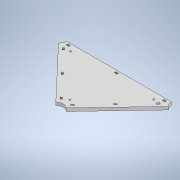
# Autodesk Inventor part: aab_face
Saved by Autodesk Inventor 2020 (Build 240168000, 168)
## iProperties
Created: 2019-09-26
Part Number: aab_face
Material: Generic
Document SubType Name: Modeling
Designer: fabrizio
Density: 1 g/cm^3
Appearance: Default
Author: fabrizio
Autodesk Inventor part; units mm, degrees
ref_plane "YZ Plane" through (0, 0, 0) normal (1, 0, 0) x (0, 1, 0)
ref_plane "XZ Plane" through (0, 0, 0) normal (0, 1, 0) x (-1, 0, 0)
ref_plane "XY Plane" through (0, 0, 0) normal (0, 0, 1) x (1, 0, 0)
sketch "Sketch1" plane through (0, 0, 0) normal (0, 1, 0) x (-1, 0, 0)
  arc A0 (10, 0) -> (6.8806, 7.2566) centre (0, 0) ccw
  arc A1 (151.2194, 7.2566) -> (148.1, 0.0154) centre (158.1, 0) ccw
  circle A2 centre (79.05, 64.475) radius 1
  circle A3 centre (133.744, 8.9222) radius 1
  circle A4 centre (24.356, 8.9222) radius 1
  line L0 (6.8806, 7.2566) -> (72.1694, 76.1134)
  line L1 (85.9306, 76.1134) -> (151.2194, 7.2566)
  line L2 (148.1, 0.0154) -> (10, 0)
  arc A5 (72.1694, 76.1134) -> (85.9306, 76.1134) centre (79.05, 83.37) ccw
  line L3 (14.0684, 2.4018) -> (17.5684, 2.4018)
  line L4 (17.5684, 2.4018) -> (17.5684, 4.4018)
  line L5 (17.5684, 4.4018) -> (14.0684, 4.4018)
  line L6 (14.0684, 4.4018) -> (14.0684, 2.4018)
  line L7 (77.3084, 2.4018) -> (80.8084, 2.4018)
  line L8 (80.8084, 2.4018) -> (80.8084, 4.4018)
  line L9 (80.8084, 4.4018) -> (77.3084, 4.4018)
  line L10 (77.3084, 4.4018) -> (77.3084, 2.4018)
  line L11 (140.5484, 2.4018) -> (144.0484, 2.4018)
  line L12 (144.0484, 2.4018) -> (144.0484, 4.4018)
  line L13 (144.0484, 4.4018) -> (140.5484, 4.4018)
  line L14 (140.5484, 4.4018) -> (140.5484, 2.4018)
  line L15 (16.2824, 8.7713) -> (18.6906, 11.3111)
  line L16 (18.6906, 11.3111) -> (17.2392, 12.6872)
  line L17 (17.2392, 12.6872) -> (14.831, 10.1474)
  line L18 (14.831, 10.1474) -> (16.2824, 8.7713)
  line L19 (43.688, 37.6746) -> (46.0962, 40.2145)
  line L20 (46.0962, 40.2145) -> (44.6449, 41.5906)
  line L21 (44.6449, 41.5906) -> (42.2367, 39.0508)
  line L22 (42.2367, 39.0508) -> (43.688, 37.6746)
  line L23 (71.0937, 66.578) -> (73.5019, 69.1178)
  line L24 (73.5019, 69.1178) -> (72.0506, 70.4939)
  line L25 (72.0506, 70.4939) -> (69.6424, 67.9541)
  line L26 (69.6424, 67.9541) -> (71.0937, 66.578)
  line L27 (143.2789, 10.1369) -> (140.8707, 12.6767)
  line L28 (140.8707, 12.6767) -> (139.4194, 11.3006)
  line L29 (139.4194, 11.3006) -> (141.8276, 8.7608)
  line L30 (141.8276, 8.7608) -> (143.2789, 10.1369)
  line L31 (115.941, 38.9688) -> (113.5329, 41.5086)
  line L32 (113.5329, 41.5086) -> (112.0815, 40.1325)
  line L33 (112.0815, 40.1325) -> (114.4897, 37.5927)
  line L34 (114.4897, 37.5927) -> (115.941, 38.9688)
  line L35 (88.6032, 67.8006) -> (86.195, 70.3404)
  line L36 (86.195, 70.3404) -> (84.7437, 68.9643)
  line L37 (84.7437, 68.9643) -> (87.1519, 66.4245)
  line L38 (87.1519, 66.4245) -> (88.6032, 67.8006)
  point P0 (148.1, 0.0154)
  point P1 (151.2194, 7.2566)
  point P2 (85.9306, 76.1134)
  constraints: 78 end point, 6 centre point, 6 point on circle
extrude "Extrusion1" add sketch "Sketch1" along normal blind 4
body "Solid1"
